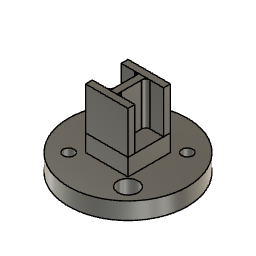
i_peg_V2 v2 (Autodesk Fusion 360 design; units mm, degrees)
Autodesk Fusion 360 part; units mm, degrees
note: some values were not read from the file. Chosen so that the rebuilt part matches the saved one: which bodies a step acts on; which face or edge a step refers to.
sketch "Sketch1" plane through (0, 0, 0) normal (0, 0, 1) x (1, 0, 0)
  line L0 (12.5, -12.5) -> (-12.5, -12.5)
  line L1 (-12.5, -12.5) -> (-12.5, 12.5)
  line L2 (-12.5, 12.5) -> (12.5, 12.5)
  line L3 (12.5, 12.5) -> (12.5, -12.5)
  line L4 (12.5, -12.5) -> (-12.5, 12.5) construction
  line L5 (-12.5, -12.5) -> (12.5, 12.5) construction
  dimension "d1" = 25
  dimension "d2" = 25
  constraint horizontal L0
  constraint perpendicular L0 L1
  constraint parallel L0 L2
  constraint parallel L1 L3
  constraint coincident L4 origin
  constraint coincident L5 origin
  measures "d1" distance of L1.end L2.end
  measures "d2" distance of L0.end L1.end
extrude "Extrude1" add sketch "Sketch1" along normal blind 10 makes body 1
sketch "Sketch2" plane through (0, 0, 10) normal (0, 0, 1) x (-1, 0, 0)
  line L0 (-12.5, -12.5) -> (12.5, -12.5)
  line L1 (12.5, -12.5) -> (12.5, 12.5)
  line L2 (12.5, 12.5) -> (-12.5, 12.5)
  line L3 (-12.5, 12.5) -> (-12.5, -12.5)
  line L4 (12.5, -12.5) -> (-12.5, -12.5)
  line L5 (-12.5, -12.5) -> (-12.5, -8.5)
  line L6 (-12.5, -8.5) -> (12.5, -8.5)
  line L7 (12.5, -8.5) -> (12.5, -12.5)
  dimension "d5" = 4
  constraint horizontal L4
  constraint vertical L5
  constraint horizontal L6
  constraint vertical L7
  constraint coincident L3 L5.end
  constraint coincident L0.end L1.start
  measures "d5" distance of L0.end L6.end
extrude "Extrude2" add sketch "Sketch2" along normal blind 25 contours L0 L1 L3 L4 L5 L6 L7 bodies 1
mirror "Mirror1" about plane through (0, 0, 0) normal (0, 1, 0) of bodies 1 merged
sketch "Sketch3" plane through (0, 0, 10) normal (0, 0, 1) x (-1, 0, 0)
  line L0 (12.5, -8.5) -> (12.5, 8.5)
  line L1 (-12.5, 8.5) -> (-12.5, -8.5)
  line L2 (-2, -8.5) -> (2, -8.5)
  line L3 (2, -8.5) -> (2, 8.5)
  line L4 (2, 8.5) -> (-2, 8.5)
  line L5 (-2, 8.5) -> (-2, -8.5)
  line L6 (-2, -8.5) -> (2, 8.5) construction
  line L7 (2, -8.5) -> (-2, 8.5) construction
  line L8 (-12.5, -8.5) -> (12.5, -8.5)
  line L9 (12.5, 8.5) -> (-12.5, 8.5)
  dimension "d10" = 4
  dimension "d11" = 17
  constraint horizontal L2
  constraint perpendicular L2 L3
  constraint parallel L2 L4
  constraint parallel L3 L5
  constraint coincident L6 origin
  constraint coincident L7 origin
  measures "d10" distance of L3.end L4.end
  measures "d11" distance of L2.end L3.end
extrude "Extrude3" add sketch "Sketch3" along normal blind 25 contours L2 L3 L4 L5 L8 L9 bodies 1
sketch "Sketch4" plane through (0, 0, 0) normal (0, 0, 1) x (1, 0, 0)
  circle A0 centre (17.5, 17.5) radius 3.25
  circle A1 centre (-17.5, -17.5) radius 3.25
  circle A2 centre (-17.5, 17.5) radius 3.25
  circle A3 centre (17.5, -17.5) radius 3.25
  circle A4 centre (0, 0) radius 35
  circle A5 centre (-17.5, 17.5) radius 6
  circle A6 centre (17.5, -17.5) radius 6
  dimension "d15" = 360
  dimension "d16" = 70
  dimension "d17" = 17.5
  dimension "d18" = 17.5
  dimension "d19" = 6.5
  dimension "d20" = 12
  dimension "d21" = 12
  constraint coincident A4.centre origin
  constraint concentric A2 A5
  constraint concentric A3 A6
  measures "d16" diameter of A4
  measures "d17" vertical distance of A4.centre A0.centre
  measures "d18" horizontal distance of A4.centre A0.centre
  measures "d19" diameter of A0
  measures "d20" diameter of A5
  measures "d21" diameter of A6
extrude "Extrude4" add sketch "Sketch4" against normal blind 10 contours A4 bodies 1
fillet "Fillet1" radius 2.5 4 edges at (-2, -8.5, 22.5) (2, -8.5, 22.5) (-2, 8.5, 22.5) (2, 8.5, 22.5) on bodies 1
split "Split1" by plane through (0, 0, 0) normal (0, 0, 1) bodies 1 makes body 2 at (4.1667, -12.5, 11.6667)
split "Split2" by plane through (0, 0, 10) normal (0, 0, 1) bodies 2 makes body 3 at (4.1667, -12.5, 18.3333)
split "Split3" by plane through (12.5, -8.5, 10) normal (0, 1, 0) bodies 3 makes body 4 at (-4.1667, 12.5, 18.3333)
split "Split4" by plane through (12.5, 8.5, 10) normal (0, -1, 0) bodies 4 makes body 5 at (2, -2, 18.3333)
split "Split5" by plane through (2, -8.5, 10) normal (1, 0, 0) and through (-2, 8.5, 10) normal (-1, 0, 0) bodies 5 makes body 6 at (2.0113, -6.2376, 18.3333) makes body 7 at (2.0028, 6.119, 18.3333) makes body 8 at (-2.0113, -6.2376, 18.3333) makes body 9 at (-2.0028, 6.119, 18.3333)
